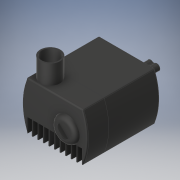
# Autodesk Inventor part: NP-600
Saved by Autodesk Inventor 2019 (Build 230136000, 136)
## iProperties
Created: 2020-10-10
Part Number: NP-600
Material: Generic
Document SubType Name: Modeling
Mass: 2608.16 g
Surface Area: 126.892 cm^2
Volume: 57.7382 cm^3
Density: 45.1721 g/cm^3
Appearance: Smooth - Black
Checked By: J. LENDI
Catalog Web Link: https://www.amazon.com/Homasy-Submersible-Aquarium-Fountain-Powerful/dp/B00EWENMAU?th=1
Description: PUMP, 80 GPH, WATER, SUBMERSIBLE, 4W
Vendor: Amazon
Author: J. LENDI
Revision Number: A
Autodesk Inventor part; units mm, degrees
ref_plane "YZ Plane" through (0, 0, 0) normal (1, 0, 0) x (0, 1, 0)
ref_plane "XZ Plane" through (0, 0, 0) normal (0, 1, 0) x (-1, 0, 0)
sketch "Sketch1" plane through (0, 0, 0) normal (0, 0, 1) x (1, 0, 0)
  line L0 (-18.161, -15.748) -> (18.161, -15.748)
  line L1 (21.336, -15.748) -> (21.336, 15.748) construction
  line L2 (18.161, 15.748) -> (-18.161, 15.748)
  line L3 (-21.336, 15.748) -> (-21.336, -15.748) construction
  line L4 (-21.336, -15.748) -> (21.336, 15.748) construction
  line L5 (21.336, -15.748) -> (-21.336, 15.748) construction
  arc A0 (-18.161, 15.748) -> (-18.161, -15.748) centre (19.3065, 0) ccw
  line L6 (-18.161, 15.748) -> (-18.161, -15.748) construction
  line L7 (-18.161, 15.748) -> (13.335, 15.748) construction
  arc A1 (18.161, -15.748) -> (18.161, 15.748) centre (-19.3065, 0) ccw
  line L8 (18.161, 15.748) -> (18.161, -15.748) construction
  line L9 (-21.336, 15.748) -> (-18.161, 15.748) construction
  line L10 (18.161, 15.748) -> (21.336, 15.748) construction
  line L11 (18.161, -15.748) -> (21.336, -15.748) construction
  line L12 (-18.161, -15.748) -> (-21.336, -15.748) construction
  point P0 (0, 0)
  dimension "d0" = 42.672
  dimension "d1" = 31.496
  dimension "d2" = 90
  dimension "d4" = 90
  dimension "d6" = 3.175
  dimension "d7" = 3.175
  constraints: 26 end point, 4 equal length, 4 point on circle, 3 horizontal, 3 perpendicular, 2 centre point, 2 midpoint, 2 tangent
  measures "d0" distance of L3.start L1.end
  measures "d1" distance of L1.end L1.start
  measures "d2" angle of L6 L7
  measures "d4" angle of L2 L8
  measures "d6" distance from line of L2.start L1
  measures "d7" distance from line of L2.end L3
extrude "Extrusion1" add sketch "Sketch1" along normal mid plane 47.498
sketch "Sketch2" plane through (-18.161, 15.748, 23.749) normal (0, 1, 0) x (1, 0, 0)
  circle A0 centre (7.62, 7.62) radius 6.477
  line L0 (0, 47.498) -> (0, 0) projected
  line L1 (36.322, 0) -> (0, 0) projected
  circle A1 centre (7.62, 7.62) radius 5.6833
  point P0 (18.161, 23.749)
  dimension "d10" = 12.954
  dimension "d11" = 7.62
  dimension "d12" = 7.62
  dimension "d13" = 0.7937
  constraints: 2 centre point
  measures "d10" diameter of A0
  measures "d11" distance from line of A0.centre L0
  measures "d12" distance from line of L1 A0.centre
  measures "d13" radial gap between concentric circles of A0 A1
extrude "Extrusion2" add sketch "Sketch2" along normal blind 12.7
ref_plane "Work Plane1" through (-10.541, 15.748, 9.652) normal (0, 0, 1) x (1, 0, 0)
split_face "Split1"
sketch "Sketch4" plane through (0, 0, 23.749) normal (0, 0, 1) x (1, 0, 0)
  circle A0 centre (8.255, 0) radius 8.255 construction
  line L0 (18.161, -15.748) -> (-18.161, -15.748) construction
  line L1 (-17.907, -15.748) -> (-14.859, -15.748)
  line L2 (-14.859, -15.748) -> (-14.859, -6.2992)
  line L3 (-14.859, -6.2992) -> (-17.907, -6.2992)
  line L4 (-17.907, -6.2992) -> (-17.907, -15.748)
  line L5 (-14.2663, -15.748) -> (-11.2183, -15.748)
  line L6 (-11.2183, -15.748) -> (-11.2183, -6.2992)
  line L7 (-11.2183, -6.2992) -> (-14.2663, -6.2992)
  line L8 (-14.2663, -6.2992) -> (-14.2663, -15.748)
  line L9 (-10.6257, -15.748) -> (-7.5777, -15.748)
  line L10 (-7.5777, -15.748) -> (-7.5777, -6.2992)
  line L11 (-7.5777, -6.2992) -> (-10.6257, -6.2992)
  line L12 (-10.6257, -6.2992) -> (-10.6257, -15.748)
  line L13 (-6.985, -15.748) -> (-3.937, -15.748)
  line L14 (-3.937, -15.748) -> (-3.937, -6.2992)
  line L15 (-3.937, -6.2992) -> (-6.985, -6.2992)
  line L16 (-6.985, -6.2992) -> (-6.985, -15.748)
  line L17 (-3.3443, -15.748) -> (-0.2963, -15.748)
  line L18 (-0.2963, -15.748) -> (-0.2963, -6.2992)
  line L19 (-0.2963, -6.2992) -> (-3.3443, -6.2992)
  line L20 (-3.3443, -6.2992) -> (-3.3443, -15.748)
  line L21 (0.2963, -15.748) -> (3.3443, -15.748)
  line L22 (3.3443, -15.748) -> (3.3443, -6.2992)
  line L23 (3.3443, -6.2992) -> (0.2963, -6.2992)
  line L24 (0.2963, -6.2992) -> (0.2963, -15.748)
  line L25 (3.937, -15.748) -> (6.985, -15.748)
  line L26 (6.985, -15.748) -> (6.985, -6.2992)
  line L27 (6.985, -6.2992) -> (3.937, -6.2992)
  line L28 (3.937, -6.2992) -> (3.937, -15.748)
  line L29 (7.5777, -15.748) -> (10.6257, -15.748)
  line L30 (10.6257, -15.748) -> (10.6257, -6.2992)
  line L31 (10.6257, -6.2992) -> (7.5777, -6.2992)
  line L32 (7.5777, -6.2992) -> (7.5777, -15.748)
  line L33 (11.2183, -15.748) -> (14.2663, -15.748)
  line L34 (14.2663, -15.748) -> (14.2663, -6.2992)
  line L35 (14.2663, -6.2992) -> (11.2183, -6.2992)
  line L36 (11.2183, -6.2992) -> (11.2183, -15.748)
  line L37 (14.859, -15.748) -> (17.907, -15.748)
  line L38 (17.907, -15.748) -> (17.907, -6.2992)
  line L39 (17.907, -6.2992) -> (14.859, -6.2992)
  line L40 (14.859, -6.2992) -> (14.859, -15.748)
  arc A1 (-18.161, 15.748) -> (-18.161, -15.748) centre (19.3065, 0) ccw construction
  line L41 (-21.336, 0) -> (21.336, 0) construction
  arc A2 (18.161, -15.748) -> (18.161, 15.748) centre (-19.3065, 0) ccw construction
  line L42 (-18.161, 15.748) -> (18.161, 15.748) construction
  line L43 (0, 15.748) -> (0, -15.748) construction
  point P0 (0, 0)
  dimension "d16" = 3.048
  dimension "d17" = 9.4488
  dimension "d18" = 0.254
  dimension "d21" = 3.6407
  dimension "d26" = 36.322
  dimension "d27" = 16.51
  dimension "d28" = 15.748
  dimension "d29" = 31.496
  constraints: 84 end point, 3 horizontal, 2 midpoint, 2 parallel, 2 point on circle, 2 point on line, 1 centre point, 1 perpendicular, 1 tangent, 72 other
  measures "d16" distance between parallel lines of L2 L4
  measures "d17" distance between parallel lines of L0 L3
  measures "d18" distance from line of L0.end L4
  measures "d21" distance of L1.start L5.start
  measures "d26" distance of L0.start L0.end
  measures "d27" diameter of A0
  measures "d28" distance between parallel lines of L0 L41
  measures "d29" distance between parallel lines of L0 L42
extrude "Extrusion3" cut sketch "Sketch4" against normal up to surface (14.097 mm away)
sketch "Sketch5" plane through (0, 0, 23.749) normal (0, 0, 1) x (1, 0, 0)
  circle A0 centre (8.255, 0) radius 8.255 projected
  point P0 (0, 0)
  constraints: 1 horizontal alignment
extrude "Extrusion4" add sketch "Sketch5" along normal blind 2.54 and the other way blind 15.5575
fillet "Fillet1" radius 3.175 1 edges at (0, 0, 26.289)
sketch "Sketch6" plane through (8.255, 0, 26.289) normal (0, 0, 1) x (1, 0, 0)
  circle A0 centre (0, 0) radius 5.08 construction
  line L0 (-3.5487, 3.635) -> (3.635, -3.5487) construction
  line L1 (-0.0228, 5.0799) -> (-0.0228, -5.0799) construction
  line L2 (2.8388, -3.4706) -> (-3.4706, 2.8388)
  line L3 (-3.4706, 2.8388) -> (-2.8388, 3.4706)
  line L4 (-2.8388, 3.4706) -> (3.4706, -2.8388)
  line L5 (3.4706, -2.8388) -> (2.8388, -3.4706)
  line L6 (2.8388, -3.4706) -> (-2.8388, 3.4706) construction
  line L7 (-3.4706, 2.8388) -> (3.4706, -2.8388) construction
  point P0 (-8.255, 0)
  dimension "d37" = 45
  constraints: 16 end point, 4 point on circle, 2 midpoint, 2 parallel, 1 perpendicular, 1 vertical
  measures "d37" angle of L1 L0
extrude "Extrusion5" add sketch "Sketch6" along normal blind 2.54
fillet "Fillet2" radius 3.175 2 edges at (5.1003, 3.1547, 28.829) (11.4097, -3.1547, 28.829)
fillet "Fillet3" radius 0.7937 11 edges at (0, 15.748, 23.749) (18.161, 15.748, 0) (18.161, -15.748, 0) (21.336, 0, 23.749) (-21.336, 0, 23.749) (-18.161, -15.748, 0) (-18.161, 15.748, 0) (0, 15.748, -23.749) (-21.336, 0, -23.749) (0, -15.748, -23.749) (21.336, 0, -23.749)
sketch "Sketch8" plane through (0, 0, -23.749) normal (0, 0, -1) x (-1, 0, 0)
  line L0 (-17.6298, 11.1442) -> (-9.3748, 11.1442) construction
  line L1 (-9.3748, 11.1442) -> (-9.3748, 14.9543) construction
  line L2 (-9.3748, 14.9543) -> (-17.6298, 14.9543) construction
  line L3 (-17.6298, 14.9543) -> (-17.6298, 11.1442) construction
  line L4 (-17.6298, 11.1442) -> (-9.3748, 14.9543) construction
  line L5 (-9.3748, 11.1442) -> (-17.6298, 14.9543) construction
  line L6 (-17.6298, 14.9543) -> (17.6298, 14.9542) construction
  circle A0 centre (-15.5661, 13.0492) radius 2.0638
  circle A1 centre (-11.4386, 13.0492) radius 2.0638
  arc A2 (-14.2885, 14.67) -> (-12.7162, 14.67) centre (-13.5023, 15.6674) ccw
  arc A3 (-12.7775, 11.4788) -> (-14.2272, 11.4788) centre (-13.5023, 10.4359) ccw
  point P0 (0, 0)
  point P1 (-13.5023, 13.0492)
  dimension "d49" = 3.81
  dimension "d50" = 8.255
  dimension "d51" = 0
  dimension "d52" = 4.1275
  dimension "d53" = 4.1275
  dimension "d57" = 1.27
  dimension "d58" = 1.27
  constraints: 12 end point, 8 point on circle, 4 centre point, 4 tangent, 2 midpoint, 2 parallel, 1 collinear, 1 horizontal, 1 perpendicular
  measures "d49" distance between parallel lines of L0 L2
  measures "d50" distance between parallel lines of L1 L3
  measures "d51" distance from line of L6.start L3
  measures "d52" diameter of A0
  measures "d53" diameter of A1
  measures "d57" radius of A3
  measures "d58" radius of A2
extrude "Extrusion6" add sketch "Sketch8" along normal blind 3.81
equation "\"d7\" = d6"
equation "\"d11\" = d12"
equation "\"d21\" = -0.222222 * d18 + 0.111111 * d26 - 0.111111 * d16"
equation "\"d28\" = 0.5 * d29"
equation "\"d57\" = d58"
body "Solid1"
